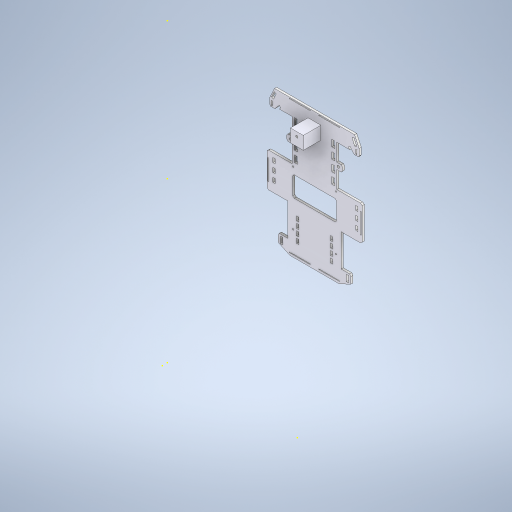
# Autodesk Inventor part: Robot_PMLD 1
Saved by Autodesk Inventor 2023 (Build 270158000, 158)
## iProperties
Created: 2025-05-12
Part Number: Robot_PMLD 1
Material: UHMW, White
Document SubType Name: Modeling
Designer: ASUS
Density: 0.94 g/cm^3
Appearance: Smooth - White
Author: ASUS
Autodesk Inventor part; units mm, degrees
ref_plane "YZ Plane" through (0, 0, 0) normal (1, 0, 0) x (0, 1, 0)
ref_plane "XZ Plane" through (0, 0, 0) normal (0, 1, 0) x (-1, 0, 0)
ref_plane "XY Plane" through (0, 0, 0) normal (0, 0, 1) x (1, 0, 0)
sketch "Sketch1" plane through (0, 0, 0) normal (0, 0, 1) x (1, 0, 0)
  line L0 (268.6934, 688.1739) -> (438.6934, 688.1739)
  line L1 (268.6934, 688.1739) -> (260.6934, 688.1739)
  line L2 (438.6934, 688.1739) -> (446.6934, 688.1739)
  line L3 (260.6934, 688.1739) -> (250.1279, 665.5162)
  line L4 (260.6934, 688.1739) -> (285.6934, 688.1739) construction
  line L5 (250.1279, 665.5162) -> (250.1279, 650.5162)
  line L6 (250.1279, 650.5162) -> (251.6279, 647.9181)
  line L7 (250.1279, 650.5162) -> (253.1279, 650.5162) construction
  line L8 (251.6279, 647.9181) -> (261.6279, 647.9181)
  line L9 (261.6279, 647.9181) -> (271.2697, 659.4088)
  line L10 (271.2697, 659.4088) -> (275.0999, 656.1948)
  line L11 (275.0999, 656.1948) -> (271.886, 652.3646)
  line L12 (271.886, 652.3646) -> (301.886, 652.3646)
  line L13 (446.6934, 688.1739) -> (457.2587, 665.5161)
  line L14 (457.2587, 665.5161) -> (457.2587, 650.5161)
  line L15 (457.2587, 650.5161) -> (455.7587, 647.9181)
  line L16 (455.7587, 647.9181) -> (445.7587, 647.9181)
  line L17 (445.7587, 647.9181) -> (436.117, 659.4088)
  line L18 (436.117, 659.4088) -> (432.2867, 656.1949)
  line L19 (432.2867, 656.1949) -> (435.5007, 652.3647)
  line L20 (435.5007, 652.3647) -> (405.5007, 652.3648)
  line L21 (301.886, 557.3687) -> (247.2816, 557.3687)
  line L22 (405.5007, 557.2878) -> (460.436, 557.2878)
  line L23 (460.436, 477.2878) -> (405.436, 477.2878)
  line L24 (405.436, 477.2878) -> (405.436, 402.2878)
  line L25 (301.6933, 402.3487) -> (271.6933, 402.3487)
  line L26 (405.436, 402.2878) -> (435.436, 402.2878)
  line L27 (435.436, 402.2878) -> (437.936, 397.9576)
  line L28 (437.936, 397.9576) -> (437.936, 382.9576)
  line L29 (271.6933, 402.3487) -> (276.6933, 402.3487) construction
  line L30 (269.3213, 397.9576) -> (269.3213, 382.9576)
  line L31 (269.3213, 382.9576) -> (296.5105, 370.2791)
  line L32 (437.936, 382.9576) -> (410.7467, 370.2791)
  line L33 (410.7467, 370.2791) -> (296.5105, 370.2791)
  line L34 (353.6934, 668.1738) -> (333.6934, 668.1738)
  line L35 (353.6934, 668.1738) -> (373.6934, 668.1738)
  line L36 (373.6934, 668.1738) -> (373.6934, 638.1738)
  line L37 (333.6934, 638.1738) -> (333.6934, 668.1738)
  line L38 (353.6934, 663.1738) -> (343.6934, 663.1738)
  line L39 (343.6934, 663.1738) -> (343.6934, 643.1738)
  line L40 (363.6934, 643.1738) -> (363.6934, 663.1738)
  line L41 (363.6934, 663.1738) -> (353.6934, 663.1738)
  line L42 (247.2816, 557.3687) -> (256.8212, 557.3687)
  line L43 (256.886, 547.3646) -> (261.886, 547.3646)
  line L44 (261.886, 547.3646) -> (261.886, 537.3646)
  line L45 (261.886, 537.3646) -> (256.886, 537.3646)
  line L46 (256.886, 537.3646) -> (256.886, 547.3646)
  line L47 (256.886, 527.3646) -> (261.886, 527.3646)
  line L48 (261.886, 527.3646) -> (261.886, 517.3646)
  line L49 (261.886, 517.3646) -> (256.886, 517.3646)
  line L50 (256.886, 517.3646) -> (256.886, 527.3646)
  line L51 (256.886, 507.3646) -> (261.886, 507.3646)
  line L52 (261.886, 507.3646) -> (261.886, 497.3646)
  line L53 (261.886, 497.3646) -> (256.886, 497.3646)
  line L54 (256.886, 497.3646) -> (256.886, 507.3646)
  line L55 (311.886, 457.3646) -> (316.886, 457.3646)
  line L56 (316.886, 457.3646) -> (316.886, 447.3646)
  line L57 (316.886, 447.3646) -> (311.886, 447.3646)
  line L58 (311.886, 447.3646) -> (311.886, 457.3646)
  line L59 (311.886, 442.3646) -> (316.886, 442.3646)
  line L60 (316.886, 442.3646) -> (316.886, 432.3646)
  line L61 (316.886, 432.3646) -> (311.886, 432.3646)
  line L62 (311.886, 432.3646) -> (311.886, 442.3646)
  line L63 (311.886, 427.3646) -> (316.886, 427.3646)
  line L64 (316.886, 427.3646) -> (316.886, 417.3646)
  line L65 (316.886, 417.3646) -> (311.886, 417.3646)
  line L66 (311.886, 417.3646) -> (311.886, 427.3646)
  line L67 (311.886, 412.3646) -> (316.886, 412.3646)
  line L68 (316.886, 412.3646) -> (316.886, 402.3646)
  line L69 (316.886, 402.3646) -> (311.886, 402.3646)
  line L70 (311.886, 402.3646) -> (311.886, 412.3646)
  line L71 (353.6286, 537.2874) -> (401.1286, 537.2874)
  line L72 (353.6286, 537.2874) -> (306.1286, 537.2874)
  line L73 (306.1286, 537.2874) -> (302.9146, 533.4572)
  line L74 (306.1286, 537.2874) -> (311.1286, 537.2874) construction
  line L75 (302.9146, 533.4572) -> (302.9146, 493.4572)
  line L76 (401.1286, 537.2874) -> (404.7816, 533.8734)
  line L77 (404.7816, 533.8734) -> (404.7816, 493.8734)
  line L78 (302.9146, 493.4572) -> (306.7497, 490.249)
  line L79 (306.7497, 490.249) -> (401.7497, 490.249)
  line L80 (401.7497, 490.249) -> (404.7816, 493.8734)
  line L81 (460.436, 557.2878) -> (450.436, 557.2878)
  line L82 (247.2816, 557.3687) -> (243.3598, 554.2673)
  line L83 (246.5737, 477.267) -> (243.3598, 481.0972)
  line L84 (246.5737, 477.267) -> (251.5737, 477.267) construction
  line L85 (243.3598, 481.0972) -> (243.3598, 554.2673)
  line L86 (460.436, 557.2878) -> (464.4205, 554.2673)
  line L87 (460.436, 477.2878) -> (464.2662, 480.5017)
  line L88 (460.436, 477.2878) -> (465.436, 477.2878) construction
  line L89 (464.2662, 480.5017) -> (464.4205, 554.2673)
  line L90 (454.4205, 547.2878) -> (449.4205, 547.2878)
  line L91 (449.4205, 547.2878) -> (449.4205, 537.2878)
  line L92 (449.4205, 537.2878) -> (454.4205, 537.2878)
  line L93 (454.4205, 537.2878) -> (454.4205, 547.2878)
  line L94 (454.4205, 527.2878) -> (449.4205, 527.2878)
  line L95 (449.4205, 527.2878) -> (449.4205, 517.2878)
  line L96 (449.4205, 517.2878) -> (454.4205, 517.2878)
  line L97 (454.4205, 517.2878) -> (454.4205, 527.2878)
  line L98 (454.4205, 507.2878) -> (449.4205, 507.2878)
  line L99 (449.4205, 507.2878) -> (449.4205, 497.2878)
  line L100 (449.4205, 497.2878) -> (454.4205, 497.2878)
  line L101 (454.4205, 497.2878) -> (454.4205, 507.2878)
  line L102 (306.886, 652.3646) -> (313.886, 652.3646)
  line L103 (313.886, 652.3646) -> (313.886, 637.3646)
  line L104 (313.886, 637.3646) -> (306.886, 637.3646)
  line L105 (306.886, 637.3646) -> (306.886, 652.3646)
  line L106 (306.886, 627.3646) -> (313.886, 627.3646)
  line L107 (313.886, 627.3646) -> (313.886, 612.3646)
  line L108 (313.886, 612.3646) -> (306.886, 612.3646)
  line L109 (306.886, 612.3646) -> (306.886, 627.3646)
  line L110 (306.886, 602.3646) -> (313.886, 602.3646)
  line L111 (313.886, 602.3646) -> (313.886, 587.3646)
  line L112 (313.886, 587.3646) -> (306.886, 587.3646)
  line L113 (306.886, 587.3646) -> (306.886, 602.3646)
  line L114 (306.886, 577.3646) -> (313.886, 577.3646)
  line L115 (313.886, 577.3646) -> (313.886, 562.3646)
  line L116 (313.886, 562.3646) -> (306.886, 562.3646)
  line L117 (306.886, 562.3646) -> (306.886, 577.3646)
  line L118 (400.5007, 652.3648) -> (393.5007, 652.3648)
  line L119 (393.5007, 652.3648) -> (393.5007, 637.3648)
  line L120 (393.5007, 637.3648) -> (400.5007, 637.3648)
  line L121 (400.5007, 637.3648) -> (400.5007, 652.3648)
  line L122 (400.5007, 627.3648) -> (393.5007, 627.3648)
  line L123 (393.5007, 627.3648) -> (393.5007, 612.3648)
  line L124 (393.5007, 612.3648) -> (400.5007, 612.3648)
  line L125 (400.5007, 612.3648) -> (400.5007, 627.3648)
  line L126 (400.5007, 602.3648) -> (393.5007, 602.3648)
  line L127 (393.5007, 602.3648) -> (393.5007, 587.3648)
  line L128 (393.5007, 587.3648) -> (400.5007, 587.3648)
  line L129 (400.5007, 587.3648) -> (400.5007, 602.3648)
  line L130 (400.5007, 577.3648) -> (393.5007, 577.3648)
  line L131 (393.5007, 577.3648) -> (393.5007, 562.3648)
  line L132 (393.5007, 562.3648) -> (400.5007, 562.3648)
  line L133 (400.5007, 562.3648) -> (400.5007, 577.3648)
  line L134 (250.1279, 665.5162) -> (255.1279, 665.5162) construction
  line L135 (253.1279, 650.5162) -> (256.1279, 650.5162)
  line L136 (256.1279, 650.5162) -> (256.1279, 660.5162)
  line L137 (256.1279, 660.5162) -> (253.1279, 660.5162)
  line L138 (253.1279, 660.5162) -> (253.1279, 650.5162)
  line L139 (452.2587, 650.5161) -> (449.2587, 650.5161)
  line L140 (449.2587, 650.5161) -> (449.2587, 660.5161)
  line L141 (449.2587, 660.5161) -> (452.2587, 660.5161)
  line L142 (452.2587, 660.5161) -> (452.2587, 650.5161)
  line L143 (258.3995, 665.5162) -> (263.3995, 665.5162) construction
  line L144 (446.991, 665.5162) -> (451.5445, 667.5814)
  line L145 (446.991, 665.5162) -> (451.5445, 667.5814)
  line L146 (451.5445, 667.5814) -> (445.3487, 681.242)
  line L147 (445.3487, 681.242) -> (440.7952, 679.1768)
  line L148 (440.7952, 679.1768) -> (446.991, 665.5162)
  line L149 (258.3995, 665.5162) -> (253.868, 667.6293)
  line L150 (258.3995, 665.5162) -> (263.3995, 665.5162) construction
  line L151 (258.3995, 665.5162) -> (253.868, 667.6293)
  line L152 (253.868, 667.6293) -> (260.2072, 681.2239)
  line L153 (260.2072, 681.2239) -> (264.7388, 679.1108)
  line L154 (264.7388, 679.1108) -> (258.3995, 665.5162)
  line L155 (269.3213, 397.9576) -> (271.6933, 402.3487)
  line L156 (274.3213, 382.9576) -> (274.3213, 397.9576)
  line L157 (274.3213, 397.9576) -> (279.3213, 397.9576)
  line L158 (279.3213, 397.9576) -> (279.3213, 382.9576)
  line L159 (279.3213, 382.9576) -> (274.3213, 382.9576)
  line L160 (432.936, 382.9576) -> (432.936, 397.9576)
  line L161 (432.936, 397.9576) -> (427.936, 397.9576)
  line L162 (427.936, 397.9576) -> (427.936, 382.9576)
  line L163 (427.936, 382.9576) -> (432.936, 382.9576)
  line L164 (343.6286, 375.2791) -> (313.6286, 375.2791)
  line L165 (313.6286, 375.2791) -> (313.6286, 380.2791)
  line L166 (313.6286, 380.2791) -> (343.6286, 380.2791)
  line L167 (343.6286, 380.2791) -> (343.6286, 375.2791)
  line L168 (363.6286, 375.2791) -> (393.6286, 375.2791)
  line L169 (393.6286, 375.2791) -> (393.6286, 380.2791)
  line L170 (393.6286, 380.2791) -> (363.6286, 380.2791)
  line L171 (363.6286, 380.2791) -> (363.6286, 375.2791)
  line L172 (301.886, 652.3646) -> (301.886, 612.3646)
  line L173 (301.886, 557.3687) -> (301.886, 597.3687)
  line L174 (301.886, 612.3646) -> (291.886, 612.3646)
  line L175 (301.886, 597.3687) -> (291.886, 597.3687)
  arc A0 (291.886, 612.3646) -> (291.886, 597.3687) centre (298.5027, 604.8667) ccw
  circle A1 centre (298.5027, 604.8667) radius 3
  line L176 (405.5007, 652.3648) -> (405.5007, 612.3648)
  line L177 (405.5007, 557.2878) -> (405.5007, 597.2878)
  line L178 (405.5007, 612.3648) -> (415.5007, 612.3648)
  line L179 (405.5007, 597.2878) -> (415.5007, 597.2878)
  arc A2 (415.5007, 597.2878) -> (415.5007, 612.3648) centre (408.9302, 604.8263) ccw
  circle A3 centre (408.9302, 604.8263) radius 3
  line L180 (301.6933, 402.3487) -> (301.6933, 477.3487)
  line L181 (301.6933, 477.3487) -> (246.5737, 477.267)
  line L182 (395.436, 457.2878) -> (390.436, 457.2878)
  line L183 (390.436, 457.2878) -> (390.436, 447.2878)
  line L184 (390.436, 447.2878) -> (395.436, 447.2878)
  line L185 (395.436, 447.2878) -> (395.436, 457.2878)
  line L186 (395.436, 442.2878) -> (390.436, 442.2878)
  line L187 (390.436, 442.2878) -> (390.436, 432.2878)
  line L188 (390.436, 432.2878) -> (395.436, 432.2878)
  line L189 (395.436, 432.2878) -> (395.436, 442.2878)
  line L190 (395.436, 427.2878) -> (390.436, 427.2878)
  line L191 (390.436, 427.2878) -> (390.436, 417.2878)
  line L192 (390.436, 417.2878) -> (395.436, 417.2878)
  line L193 (395.436, 417.2878) -> (395.436, 427.2878)
  line L194 (395.436, 412.2878) -> (390.436, 412.2878)
  line L195 (390.436, 412.2878) -> (390.436, 402.2878)
  line L196 (390.436, 402.2878) -> (395.436, 402.2878)
  line L197 (395.436, 402.2878) -> (395.436, 412.2878)
  line L198 (343.6934, 643.1738) -> (343.6934, 638.1738)
  line L199 (363.6934, 643.1738) -> (363.6934, 638.1738)
  line L200 (333.6934, 638.1738) -> (343.6934, 638.1738)
  line L201 (363.6934, 638.1738) -> (373.6934, 638.1738)
  line L202 (401.7497, 490.249) -> (398.7497, 490.249)
  line L203 (306.7497, 490.249) -> (309.7497, 490.249)
  circle A4 centre (403.2657, 467.0612) radius 1.6
  circle A5 centre (303.4357, 467.0612) radius 1.6
  circle A6 centre (303.4357, 593.0112) radius 1.6
  circle A7 centre (403.2657, 593.0112) radius 1.6
  point P0 (0, 0)
  dimension "d0" = 170
  dimension "d1" = 8
  dimension "d2" = 8
  dimension "d3" = 25
  dimension "d4" = 115
  dimension "d5" = 15
  dimension "d11" = 3
  dimension "d12" = 60
  dimension "d13" = 10
  dimension "d14" = 15
  dimension "d15" = 130
  dimension "d16" = 5
  dimension "d17" = 5
  dimension "d19" = 30
  dimension "d22" = 25
  dimension "d23" = 15
  dimension "d27" = 3
  dimension "d28" = 10
  dimension "d29" = 15
  dimension "d30" = 130
  dimension "d31" = 5
  dimension "d32" = 5
  dimension "d33" = 30
  dimension "d47" = 55
  dimension "d51" = 75
  dimension "d52" = 30
  dimension "d53" = 30
  dimension "d54" = 5
  dimension "d55" = 120
  dimension "d56" = 15
  dimension "d59" = 15
  dimension "d60" = 30
  dimension "d61" = 115
  dimension "d62" = 30
  dimension "d75" = 30
  dimension "d76" = 40
  dimension "d77" = 5
  dimension "d78" = 10
  dimension "d79" = 20
  dimension "d81" = 20
  dimension "d82" = 10
  dimension "d100" = 5
  dimension "d101" = 10
  dimension "d103" = 5
  dimension "d104" = 10
  dimension "d106" = 5
  dimension "d107" = 10
  dimension "d113" = 5
  dimension "d114" = 10
  dimension "d116" = 5
  dimension "d117" = 10
  dimension "d119" = 5
  dimension "d120" = 10
  dimension "d122" = 5
  dimension "d123" = 10
  dimension "d139" = 5
  dimension "d140" = 130
  dimension "d141" = 40
  dimension "d142" = 5
  dimension "d143" = 40
  dimension "d144" = 5
  dimension "d145" = 95
  dimension "d147" = 5
  dimension "d148" = 5
  constraints: 408 end point, 61 parallel, 54 horizontal, 38 perpendicular, 8 centre point, 8 vertical, 7 point on line, 6 equal length, 4 point on circle, 3 collinear, 2 coincident
  measures "d0" distance of L0.start L0.end
  measures "d1" distance of L0.start L1.end
  measures "d2" distance of L0.end L2.end
  measures "d3" distance of L1.end L3.end
  measures "d4" angle of L3 L4
  measures "d5" distance of L3.end L5.end
  measures "d11" distance of L5.end L6.end
  measures "d12" angle of L6 L7
  measures "d13" distance of L6.end L8.end
  measures "d14" distance of L8.end L9.end
  measures "d15" angle of L9 L8
  measures "d16" distance of L9.end L10.end
  measures "d17" distance of L10.end L11.end
  measures "d19" distance of L11.end L12.end
  measures "d22" distance of L2.end L13.end
  measures "d23" distance of L13.end L14.end
  measures "d27" distance of L14.end L15.end
  measures "d28" distance of L15.end L16.end
  measures "d29" distance of L16.end L17.end
  measures "d30" angle of L16 L17
  measures "d31" distance of L17.end L18.end
  measures "d32" distance of L18.end L19.end
  measures "d33" distance of L19.end L20.end
  measures "d47" distance of L23.start L23.end
  measures "d51" distance of L23.end L24.end
  measures "d52" distance of L25.start L25.end
  measures "d53" distance of L24.end L26.end
  measures "d54" distance of L26.end L27.end
  measures "d55" angle of L26 L27
  measures "d56" distance of L27.end L28.end
  measures "d59" distance of L30.start L30.end
  measures "d60" distance of L30.end L31.end
  measures "d61" angle of L31 L30
  measures "d62" distance of L28.end L32.end
  measures "d75" distance of L35.end L36.end
  measures "d76" distance of L36.end L37.start
  measures "d77" distance of L34.start L38.start
  measures "d78" distance of L38.start L38.end
  measures "d79" distance of L38.end L39.end
  measures "d81" distance of L40.start L40.end
  measures "d82" distance of L40.end L38.start
  measures "d100" distance of L44.end L45.end
  measures "d101" distance of L43.end L44.end
  measures "d103" distance of L48.end L49.end
  measures "d104" distance of L47.end L48.end
  measures "d106" distance of L52.end L53.end
  measures "d107" distance of L51.end L52.end
  measures "d113" distance of L56.end L57.end
  measures "d114" distance of L55.end L56.end
  measures "d116" distance of L60.end L61.end
  measures "d117" distance of L59.end L60.end
  measures "d119" distance of L64.end L65.end
  measures "d120" distance of L63.end L64.end
  measures "d122" distance of L68.end L69.end
  measures "d123" distance of L67.end L68.end
  measures "d139" distance of L72.end L73.end
  measures "d140" angle of L73 L74
  measures "d141" distance of L73.end L75.end
  measures "d142" distance of L71.end L76.end
  measures "d143" distance of L76.end L77.end
  measures "d144" distance of L75.end L78.end
  measures "d145" distance of L78.end L79.end
  measures "d147" distance of L21.end L82.end
  measures "d148" distance of L83.start L83.end
sketch "Sketch2" plane through (0, 0, 0) normal (0, 0, 1) x (1, 0, 0)
  point P0 (0, 0)
sketch "Sketch5" plane through (0, 0, 0) normal (0, 0, 1) x (1, 0, 0)
  point P0 (0, 0)
extrude "Extrusion5" add sketch "Sketch1" along normal blind 50 contours L35 L36 L201 L199 L40 L41 L38 L39 L198 L200 L37 L34
extrude "Extrusion6" add sketch "Sketch1" along normal blind 12 contours L0 L2 L13 L14 L15 L16 L17 L18 L19 L20 L176 L178 A2 L179 L177 L22 L86 L89 L87 L23 L24 L26 L27 L28 L32 L33 L31 L30 L155 L25 L180 L181 L83 L85 L82 L21 L173 A6 L175 A0 L174 L172 L12 L11 L10 L9 L8 L6 L5 L3 L1 | A6 L173 | A4 | A5 | A7 picked at (302.9218, 592.6447)
sketch "Sketch13" plane through (0, 0, 12) normal (0, 0, 1) x (1, 0, 0)
  point P0 (0, 0)
sketch "Sketch14" plane through (0, 0, 12) normal (0, 0, 1) x (1, 0, 0)
  point P0 (0, 0)
sketch "Sketch15" plane through (0, 0, 12) normal (0, 0, 1) x (1, 0, 0)
  point P0 (0, 0)
sketch "Sketch16" plane through (301.886, 557.3687, 0) normal (-1, 0, 0) x (0, 0, 1)
  point P0 (0, -557.3687)
sketch "Sketch17" plane through (0, 0, 12) normal (0, 0, 1) x (1, 0, 0)
  point P0 (0, 0)
thread "Thread1" size "M6x1" class "6H" standard "ANSI Metric M Profile" length 43.6
thread "Thread2" size "M6x1" class "6H" standard "ANSI Metric M Profile" length 43.6
sketch "Sketch18" plane through (0, 0, 12) normal (0, 0, 1) x (1, 0, 0)
  point P0 (0, 0)
sketch "Sketch19" plane through (0, 0, 12) normal (0, 0, 1) x (1, 0, 0)
  point P0 (0, 0)
sketch "Sketch24" plane through (301.6933, 402.3487, 0) normal (-1, 0, 0) x (0, 0, 1)
  point P0 (0, -402.3487)
sketch "Sketch26" plane through (301.6933, 402.3487, 0) normal (-1, 0, 0) x (0, 0, 1)
  point P0 (0, -402.3487)
sketch "Sketch27" plane through (301.6933, 477.3487, 0) normal (0.0014818, -0.9999989, 0) x (0.9999989, 0.0014818, 0)
  line L0 (0, 0) -> (-0.1111, 0) projected
  line L1 (0, 0) -> (-10, 0)
  line L2 (-55.1196, 0) -> (0, 0) projected
  line L3 (-10, 0) -> (-10, 12)
  line L4 (100.0754, 0) -> (5.0755, 0) projected
  line L5 (-10, 0) -> (2, 0) construction
  line L6 (-55.1196, 12) -> (0, 12) projected
  line L7 (-10, 12) -> (0, 12)
  line L8 (0, 12) -> (0, 0)
  point P0 (-302.4003, 0)
  dimension "d332" = 10
  dimension "d333" = 12
  dimension "d334" = 90
  dimension "d335" = 10
  dimension "d336" = 12
  constraints: 10 end point, 2 perpendicular, 1 horizontal, 1 point on line
  measures "d332" distance of L0.start L1.end
  measures "d333" distance of L1.end L3.end
  measures "d334" angle of L5 L3
  measures "d335" distance of L3.end L6.end
  measures "d336" distance of L6.end L0.start
extrude "Extrusion16" add sketch "Sketch27" along normal blind 75
sketch "Sketch28" plane through (405.436, 477.2878, 0) normal (0, -1, 0) x (1, 0, 0)
  line L0 (0, 0) -> (0, 12) projected
  line L1 (0, 0) -> (10, 0)
  line L2 (0, 0) -> (55, 0) projected
  line L3 (10, 0) -> (10, 12)
  line L4 (0, 12) -> (55, 12) projected
  line L5 (10, 12) -> (0, 12)
  line L6 (0, 12) -> (0, 0)
  point P0 (-405.436, 0)
  dimension "d339" = 10
  dimension "d340" = 12
  dimension "d341" = 90
  dimension "d342" = 10
  dimension "d343" = 12
  constraints: 8 end point, 2 perpendicular, 1 point on line
  measures "d339" distance of L0.start L1.end
  measures "d340" distance of L1.end L3.end
  measures "d341" angle of L3 L1
  measures "d342" distance of L3.end L5.end
  measures "d343" distance of L5.end L0.start
extrude "Extrusion17" add sketch "Sketch28" along normal blind 75
sketch "Sketch29" plane through (0, 0, 12) normal (0, 0, 1) x (1, 0, 0)
  point P0 (0, 0)
sketch "Sketch30" plane through (0, 0, 12) normal (0, 0, 1) x (1, 0, 0)
  line L0 (302.9146, 533.4572) -> (306.1286, 537.2874) projected
  line L1 (306.1286, 537.2874) -> (401.1286, 537.2874) projected
  circle A0 centre (303.7136, 552.2874) radius 1.6
  circle A1 centre (403.5436, 552.2874) radius 1.6
  line L2 (405.5007, 557.2878) -> (405.5007, 597.2878) projected
  circle A2 centre (403.5436, 426.3374) radius 1.6
  circle A3 centre (303.7136, 426.3374) radius 1.6
  point P0 (0, 0)
  dimension "d351" = 3.2
  dimension "d352" = 3.2
  dimension "d355" = 3.2
  dimension "d357" = 3.2
  constraints: 4 centre point
  measures "d351" diameter of A0
  measures "d352" diameter of A1
  measures "d355" diameter of A2
  measures "d357" diameter of A3
extrude "Extrusion18" cut sketch "Sketch30" against normal blind 20 contours A3
extrude "Extrusion19" cut sketch "Sketch30" against normal blind 20 contours A2
extrude "Extrusion20" cut sketch "Sketch30" against normal blind 20 contours A1
extrude "Extrusion21" cut sketch "Sketch30" against normal blind 20 contours A0
thread "Thread7" size "M3.5x0.6" class "6H" standard "ANSI Metric M Profile" length 43.6
thread "Thread8" size "M3.5x0.6" class "6H" standard "ANSI Metric M Profile" length 43.6
thread "Thread9" size "M3.5x0.6" class "6H" standard "ANSI Metric M Profile" length 43.6
thread "Thread10" size "M3.5x0.6" class "6H" standard "ANSI Metric M Profile" length 43.6
sketch "Sketch31" plane through (0, 0, 50) normal (0, 0, 1) x (1, 0, 0)
  line L0 (333.6934, 638.1738) -> (343.6934, 638.1738) projected
  line L1 (333.6934, 668.1738) -> (333.6934, 638.1738) projected
  line L2 (333.6934, 638.1738) -> (333.6934, 668.1738)
  line L3 (373.6934, 668.1738) -> (333.6934, 668.1738) projected
  line L4 (333.6934, 668.1738) -> (373.6934, 668.1738)
  line L5 (373.6934, 638.1738) -> (373.6934, 668.1738) projected
  line L6 (373.6934, 668.1738) -> (373.6934, 638.1738)
  line L7 (373.6934, 638.1738) -> (333.6934, 638.1738)
  point P0 (0, 0)
  dimension "d374" = 30
  dimension "d375" = 40
  dimension "d376" = 30
  dimension "d377" = 40
  constraints: 8 end point, 2 collinear, 2 perpendicular
  measures "d374" distance of L0.start L1.start
  measures "d375" distance of L1.start L3.start
  measures "d376" distance of L3.start L5.start
  measures "d377" distance of L5.start L0.start
extrude "Extrusion22" add sketch "Sketch31" along normal blind 3
sketch "Sketch32" plane through (0, 0, 53) normal (0, 0, 1) x (1, 0, 0)
  line L0 (373.6934, 668.1738) -> (333.6934, 668.1738) projected
  circle A0 centre (353.6934, 658.1738) radius 2.5
  point P0 (0, 0)
  dimension "d381" = 5
  constraints: 1 centre point
  measures "d381" diameter of A0
extrude "Extrusion23" cut sketch "Sketch32" against normal blind 2
thread "Thread11" size "M5x0.8" class "6H" standard "ANSI Metric M Profile" length 43.6
sketch "Sketch33" plane through (0, 0, 12) normal (0, 0, 1) x (1, 0, 0)
  line L0 (296.5105, 370.2791) -> (410.7467, 370.2791) projected
  line L1 (313.6286, 375.2791) -> (313.6286, 380.2791) projected
  line L2 (313.6286, 375.2791) -> (295.6286, 375.2791)
  line L3 (295.6286, 375.2791) -> (295.6286, 380.2791)
  line L4 (295.6286, 380.2791) -> (313.6286, 380.2791)
  line L5 (393.6286, 380.2791) -> (393.6286, 375.2791) projected
  line L6 (393.6286, 380.2791) -> (411.6286, 380.2791)
  line L7 (411.6286, 380.2791) -> (411.6286, 375.2791)
  line L8 (411.6286, 375.2791) -> (393.6286, 375.2791)
  point P0 (0, 0)
  dimension "d388" = 18
  dimension "d389" = 5
  dimension "d390" = 18
  dimension "d391" = 5
  dimension "d392" = 18
  constraints: 12 end point, 2 horizontal, 1 perpendicular, 1 vertical
  measures "d388" distance of L1.start L2.end
  measures "d389" distance of L2.end L3.end
  measures "d390" distance of L5.start L6.end
  measures "d391" distance of L6.end L7.end
  measures "d392" distance of L7.end L5.end
extrude "Extrusion24" cut sketch "Sketch33" against normal blind 20 contours L2 L3 L4 L1
extrude "Extrusion25" cut sketch "Sketch33" against normal blind 20 contours L6 L7 L8 L5
sketch "Sketch34" plane through (0, 0, 12) normal (0, 0, 1) x (1, 0, 0)
  point P0 (0, 0)
sketch "Sketch35" plane through (0, 0, 12) normal (0, 0, 1) x (1, 0, 0)
  line L0 (343.6286, 380.2791) -> (343.6286, 375.2791) projected
  line L1 (343.6286, 375.2791) -> (343.6286, 376.7791)
  line L2 (343.6286, 376.7791) -> (295.6286, 376.7791)
  line L3 (295.6286, 380.2791) -> (295.6286, 375.2791) projected
  line L4 (295.6286, 376.7791) -> (295.6286, 380.2791)
  line L5 (295.6286, 380.2791) -> (343.6286, 380.2791) projected
  line L6 (295.6286, 380.2791) -> (343.6286, 380.2791)
  line L7 (343.6286, 380.2791) -> (343.6286, 376.7791)
  line L8 (411.6286, 375.2791) -> (363.6286, 375.2791) projected
  line L9 (411.6286, 375.2791) -> (411.6286, 376.7791)
  line L10 (411.6286, 380.2791) -> (411.6286, 375.2791) projected
  line L11 (411.6286, 376.7791) -> (363.6286, 376.7791)
  line L12 (363.6286, 380.2791) -> (411.6286, 380.2791) projected
  line L13 (363.6286, 376.7791) -> (363.6286, 380.2791)
  line L14 (363.6286, 380.2791) -> (411.6286, 380.2791)
  line L15 (411.6286, 380.2791) -> (411.6286, 376.7791)
  point P0 (0, 0)
  dimension "d397" = 1.5
  dimension "d398" = 48
  dimension "d399" = 3.5
  dimension "d400" = 48
  dimension "d401" = 3.5
  dimension "d402" = 1.5
  dimension "d403" = 48
  dimension "d404" = 3.5
  dimension "d405" = 48
  dimension "d406" = 3.5
  constraints: 20 end point, 4 perpendicular, 2 collinear, 2 point on line
  measures "d397" distance of L0.end L1.end
  measures "d398" distance of L1.end L2.end
  measures "d399" distance of L2.end L3.start
  measures "d400" distance of L3.start L0.start
  measures "d401" distance of L0.start L1.end
  measures "d402" distance of L8.start L9.end
  measures "d403" distance of L9.end L11.end
  measures "d404" distance of L11.end L12.start
  measures "d405" distance of L12.start L10.start
  measures "d406" distance of L10.start L9.end
sketch "Sketch36" plane through (296.5105, 370.2791, 0) normal (0, -1, 0) x (1, 0, 0)
  point P0 (-296.5105, 0)
extrude "Extrusion26" add sketch "Sketch35" against normal blind 12 contours L0 L2 L3 L5
extrude "Extrusion27" add sketch "Sketch35" against normal blind 12 contours L10 L11 L13 L12
sketch "Sketch37" plane through (0, 0, 12) normal (0, 0, 1) x (1, 0, 0)
  line L0 (446.6934, 688.1739) -> (260.6934, 688.1739) projected
  line L1 (343.6934, 686.1739) -> (295.6934, 686.1739)
  line L2 (295.6934, 686.1739) -> (295.6934, 684.6739)
  line L3 (295.6934, 684.6739) -> (343.6934, 684.6739)
  line L4 (343.6934, 684.6739) -> (343.6934, 686.1739)
  line L5 (363.6934, 686.1739) -> (411.6934, 686.1739)
  line L6 (411.6934, 686.1739) -> (411.6934, 684.6739)
  line L7 (411.6934, 684.6739) -> (363.6934, 684.6739)
  line L8 (363.6934, 684.6739) -> (363.6934, 686.1739)
  point P0 (0, 0)
  dimension "d415" = 48
  dimension "d416" = 1.5
  dimension "d417" = 48
  dimension "d418" = 1.5
  dimension "d420" = 48
  dimension "d421" = 1.5
  dimension "d422" = 48
  dimension "d423" = 1.5
  constraints: 16 end point, 2 horizontal, 2 parallel, 1 perpendicular, 1 vertical
  measures "d415" distance of L1.start L1.end
  measures "d416" distance of L1.end L2.end
  measures "d417" distance of L2.end L3.end
  measures "d418" distance of L3.end L1.start
  measures "d420" distance of L5.start L5.end
  measures "d421" distance of L5.end L6.end
  measures "d422" distance of L6.end L7.end
  measures "d423" distance of L7.end L5.start
extrude "Extrusion28" cut sketch "Sketch37" against normal blind 12 contours L4 L3 L2 L1
extrude "Extrusion29" cut sketch "Sketch37" against normal blind 12 contours L5 L6 L7 L8
sketch "Sketch38" plane through (0, 0, 12) normal (0, 0, 1) x (1, 0, 0)
  line L0 (243.3598, 554.2673) -> (243.3598, 481.0972) projected
  line L1 (245.3598, 517.6823) -> (245.3598, 541.6823)
  line L2 (245.3598, 541.6823) -> (246.8598, 541.6823)
  line L3 (246.8598, 541.6823) -> (246.8598, 493.6823)
  line L4 (246.8598, 493.6823) -> (245.3598, 493.6823)
  line L5 (245.3598, 493.6823) -> (245.3598, 517.6823)
  point P0 (0, 0)
  dimension "d429" = 24
  dimension "d430" = 1.5
  dimension "d431" = 48
  dimension "d432" = 1.5
  dimension "d433" = 24
  constraints: 10 end point, 2 perpendicular, 1 collinear, 1 point on line
  measures "d429" distance of L1.start L1.end
  measures "d430" distance of L1.end L2.end
  measures "d431" distance of L2.end L3.end
  measures "d432" distance of L3.end L4.end
  measures "d433" distance of L4.end L1.start
extrude "Extrusion30" cut sketch "Sketch38" against normal blind 12
sketch "Sketch39" plane through (0, 0, 12) normal (0, 0, 1) x (1, 0, 0)
  line L0 (464.2662, 480.5017) -> (464.4205, 554.2673) projected
  line L1 (462.3434, 517.3845) -> (462.3434, 541.3845)
  line L2 (462.3434, 541.3845) -> (460.8434, 541.3845)
  line L3 (460.8434, 541.3845) -> (460.8434, 493.3845)
  line L4 (460.8434, 493.3845) -> (462.3434, 493.3845)
  line L5 (462.3434, 493.3845) -> (462.3434, 517.3845)
  point P0 (0, 0)
  dimension "d437" = 24
  dimension "d438" = 1.5
  dimension "d439" = 48
  dimension "d440" = 1.5
  dimension "d441" = 24
  constraints: 10 end point, 2 perpendicular, 1 point on line
  measures "d437" distance of L1.start L1.end
  measures "d438" distance of L1.end L2.end
  measures "d439" distance of L2.end L3.end
  measures "d440" distance of L3.end L4.end
  measures "d441" distance of L4.end L1.start
extrude "Extrusion31" cut sketch "Sketch39" against normal blind 12
sketch "Sketch40" plane through (333.6934, 668.1738, 12) normal (0, 1, 0) x (1, 0, 0)
  line L0 (40, 0) -> (40, -41) projected
  line L1 (78, 0) -> (30, 0) projected
  line L2 (40, -41) -> (38, -41)
  line L3 (38, -41) -> (38, 0)
  line L4 (38, 0) -> (40, 0)
  line L5 (40, 0) -> (40, -41)
  line L6 (0, 0) -> (0, -41) projected
  line L7 (10, 0) -> (-38, 0) projected
  line L8 (0, -41) -> (2, -41)
  line L9 (2, -41) -> (2, 0)
  line L10 (2, 0) -> (0, 0)
  line L11 (0, 0) -> (0, -41)
  point P0 (-333.6934, 12)
  dimension "d444" = 2
  dimension "d445" = 2
  constraints: 16 end point, 4 parallel, 2 horizontal, 2 perpendicular, 2 point on line
  measures "d444" distance of L3.end L4.end
  measures "d445" distance of L10.end L9.end
extrude "Extrusion32" cut sketch "Sketch40" against normal blind 100
sketch "Sketch41" plane through (335.6934, 668.1738, 53) normal (0, 1, 0) x (1, 0, 0)
  line L0 (36, 0) -> (36, 41) projected
  line L1 (111, 41) -> (-75, 41) projected
  line L2 (36, 0) -> (33, 0)
  line L3 (33, 0) -> (33, 41)
  line L4 (33, 41) -> (36, 41)
  line L5 (36, 41) -> (36, 0)
  line L6 (0, 41) -> (0, 0) projected
  line L7 (0, 0) -> (3, 0)
  line L8 (3, 0) -> (3, 41)
  line L9 (3, 41) -> (0, 41)
  line L10 (0, 41) -> (0, 0)
  point P0 (-335.6934, 53)
  point P1 (3, 41)
  dimension "d448" = 3
  dimension "d449" = 3
  constraints: 16 end point, 4 parallel, 2 horizontal, 2 perpendicular, 2 point on line
  measures "d448" distance of L3.end L4.end
  measures "d449" distance of L9.end L8.end
extrude "Extrusion33" cut sketch "Sketch41" against normal blind 100
sketch "Sketch42" plane through (0, 0, 12) normal (0, 0, 1) x (1, 0, 0)
  point P0 (0, 0)
sketch "Sketch43" plane through (260.6934, 688.1739, 0) normal (0, 1, 0) x (1, 0, 0)
  point P0 (-260.6934, 0)
sketch "Sketch44" plane through (0, 0, 0) normal (0, 0, -1) x (-1, 0, 0)
  line L0 (-446.6934, 688.1739) -> (-260.6934, 688.1739) projected
  line L1 (-446.6934, 688.1739) -> (-260.6934, 688.1739)
  line L2 (-250.1279, 665.5162) -> (-250.1279, 650.5162) projected
  line L3 (-260.6934, 688.1739) -> (-250.1279, 665.5162)
  line L4 (-250.1279, 665.5162) -> (-250.1279, 650.5162)
  line L5 (-250.1279, 650.5162) -> (-251.6279, 647.9181) projected
  line L6 (-250.1279, 650.5162) -> (-251.6279, 647.9181)
  line L7 (-261.6279, 647.9181) -> (-271.2697, 659.4088) projected
  line L8 (-251.6279, 647.9181) -> (-261.6279, 647.9181)
  line L9 (-261.6279, 647.9181) -> (-271.2697, 659.4088)
  line L10 (-275.0999, 656.1948) -> (-271.886, 652.3646) projected
  line L11 (-271.2697, 659.4088) -> (-275.0999, 656.1948)
  line L12 (-275.0999, 656.1948) -> (-271.886, 652.3646)
  line L13 (-271.886, 652.3646) -> (-301.886, 652.3646) projected
  line L14 (-271.886, 652.3646) -> (-301.886, 652.3646)
  line L15 (-301.886, 652.3646) -> (-301.886, 612.3646) projected
  line L16 (-301.886, 652.3646) -> (-301.886, 612.3646)
  line L17 (-301.886, 612.3646) -> (-291.886, 612.3646) projected
  line L18 (-301.886, 612.3646) -> (-291.886, 612.3646)
  line L19 (-291.886, 597.3687) -> (-301.886, 597.3687) projected
  arc A0 (-291.886, 597.3687) -> (-291.886, 612.3646) centre (-298.5027, 604.8667) ccw
  line L20 (-291.886, 597.3687) -> (-301.886, 597.3687)
  line L21 (-301.886, 557.3687) -> (-247.2816, 557.3687) projected
  line L22 (-301.886, 597.3687) -> (-301.886, 557.3687)
  line L23 (-457.2587, 665.5161) -> (-446.6934, 688.1739) projected
  line L24 (-446.6934, 688.1739) -> (-457.2587, 665.5161)
  line L25 (-457.2587, 650.5161) -> (-457.2587, 665.5161) projected
  line L26 (-457.2587, 665.5161) -> (-457.2587, 650.5161)
  line L27 (-445.7587, 647.9181) -> (-455.7587, 647.9181) projected
  line L28 (-457.2587, 650.5161) -> (-455.7587, 647.9181)
  line L29 (-455.7587, 647.9181) -> (-445.7587, 647.9181)
  line L30 (-432.2867, 656.1949) -> (-436.117, 659.4088) projected
  line L31 (-445.7587, 647.9181) -> (-436.117, 659.4088)
  line L32 (-436.117, 659.4088) -> (-432.2867, 656.1949)
  line L33 (-405.5007, 652.3648) -> (-435.5007, 652.3647) projected
  line L34 (-432.2867, 656.1949) -> (-435.5007, 652.3647)
  line L35 (-435.5007, 652.3647) -> (-405.5007, 652.3647)
  line L36 (-405.5007, 612.3648) -> (-405.5007, 652.3648) projected
  line L37 (-405.5007, 652.3647) -> (-405.5007, 612.3647)
  line L38 (-405.5007, 612.3647) -> (-415.5007, 612.3648)
  line L39 (-415.5007, 612.3648) -> (-405.5007, 612.3648) projected
  line L40 (-405.5007, 597.2878) -> (-415.5007, 597.2878) projected
  arc A1 (-415.5007, 612.3648) -> (-415.5007, 597.2878) centre (-408.9302, 604.8263) ccw
  line L41 (-415.5007, 597.2878) -> (-405.5007, 597.2878)
  line L42 (-405.5007, 557.2878) -> (-405.5007, 597.2878) projected
  line L43 (-405.5007, 597.2878) -> (-405.5007, 557.2878)
  line L44 (-464.4205, 554.2673) -> (-460.436, 557.2878) projected
  line L45 (-405.5007, 557.2878) -> (-460.436, 557.2878)
  line L46 (-460.436, 557.2878) -> (-464.4205, 554.2673)
  line L47 (-460.436, 477.2878) -> (-464.2662, 480.5017) projected
  line L48 (-464.4205, 554.2673) -> (-464.2662, 480.5017)
  line L49 (-464.2662, 480.5017) -> (-460.436, 477.2878)
  line L50 (-415.436, 477.2878) -> (-415.436, 402.2878) projected
  line L51 (-460.436, 477.2878) -> (-415.436, 477.2878)
  line L52 (-415.436, 477.2878) -> (-415.436, 402.2878)
  line L53 (-435.436, 402.2878) -> (-415.436, 402.2878) projected
  line L54 (-415.436, 402.2878) -> (-435.436, 402.2878)
  line L55 (-437.936, 397.9576) -> (-435.436, 402.2878) projected
  line L56 (-435.436, 402.2878) -> (-437.936, 397.9576)
  line L57 (-437.936, 382.9576) -> (-437.936, 397.9576) projected
  line L58 (-437.936, 397.9576) -> (-437.936, 382.9576)
  line L59 (-296.5105, 370.2791) -> (-410.7467, 370.2791) projected
  line L60 (-437.936, 382.9576) -> (-410.7467, 370.2791)
  line L61 (-269.3213, 382.9576) -> (-296.5105, 370.2791) projected
  line L62 (-410.7467, 370.2791) -> (-296.5105, 370.2791)
  line L63 (-269.3213, 397.9576) -> (-269.3213, 382.9576) projected
  line L64 (-296.5105, 370.2791) -> (-269.3213, 382.9576)
  line L65 (-269.3213, 382.9576) -> (-269.3213, 397.9576)
  line L66 (-271.6933, 402.3487) -> (-269.3213, 397.9576) projected
  line L67 (-269.3213, 397.9576) -> (-271.6933, 402.3487)
  line L68 (-291.8044, 402.3487) -> (-271.6933, 402.3487) projected
  line L69 (-271.6933, 402.3487) -> (-291.8044, 402.3487)
  line L70 (-291.8044, 402.3487) -> (-291.8044, 477.3487)
  line L71 (-246.5737, 477.267) -> (-291.6933, 477.3339) projected
  line L72 (-291.8044, 477.3487) -> (-246.5737, 477.267)
  line L73 (-243.3598, 554.2673) -> (-243.3598, 481.0972) projected
  line L74 (-246.5737, 477.267) -> (-243.3598, 481.0972)
  line L75 (-243.3598, 481.0972) -> (-243.3598, 554.2673)
  line L76 (-247.2816, 557.3687) -> (-243.3598, 554.2673) projected
  line L77 (-243.3598, 554.2673) -> (-247.2816, 557.3687)
  line L78 (-247.2816, 557.3687) -> (-301.886, 557.3687)
  point P0 (0, 0)
  dimension "d452" = 10
  dimension "d453" = 15
  dimension "d454" = 5
  dimension "d455" = 5
  dimension "d456" = 30
  dimension "d457" = 40
  dimension "d458" = 10
  dimension "d459" = 10
  dimension "d460" = 10
  dimension "d461" = 40
  dimension "d462" = 25
  dimension "d463" = 15
  dimension "d464" = 3
  dimension "d465" = 10
  dimension "d466" = 15
  dimension "d467" = 5
  dimension "d468" = 5
  dimension "d469" = 30
  dimension "d470" = 40
  dimension "d471" = 10
  dimension "d472" = 10
  dimension "d473" = 10
  dimension "d474" = 40
  dimension "d475" = 75
  constraints: 93 end point, 19 collinear, 11 perpendicular, 8 parallel, 4 point on circle, 2 centre point, 1 point on line
  measures "d452" distance of L5.end L7.start
  measures "d453" distance of L7.start L7.end
  measures "d454" distance of L7.end L10.start
  measures "d455" distance of L10.start L10.end
  measures "d456" distance of L10.end L13.end
  measures "d457" distance of L13.end L15.end
  measures "d458" distance of L15.end L17.end
  measures "d459" radius of A0
  measures "d460" distance of L19.start L19.end
  measures "d461" distance of L19.end L21.start
  measures "d462" distance of L0.start L23.start
  measures "d463" distance of L23.start L25.start
  measures "d464" distance of L25.start L27.end
  measures "d465" distance of L27.end L27.start
  measures "d466" distance of L27.start L30.end
  measures "d467" distance of L30.end L30.start
  measures "d468" distance of L30.start L33.end
  measures "d469" distance of L33.end L35.end
  measures "d470" distance of L35.end L37.end
  measures "d471" distance of L37.end L38.end
  measures "d472" radius of A1
  measures "d473" distance of L40.end L40.start
  measures "d474" distance of L40.start L42.start
  measures "d475" distance of L68.start L70.end
extrude "Extrusion34" cut sketch "Sketch44" against normal blind 7
sketch "Sketch45" plane through (291.6933, 477.3339, 0) normal (-0.9999989, -0.0014818, 0) x (0, 0, 1)
  line L0 (7, 0) -> (12, 0) projected
  line L1 (12, 0) -> (7, 0)
  line L2 (7, 0) -> (7, -75)
  line L3 (7, -75) -> (12, -75)
  line L4 (12, -75) -> (12, 0)
  line L5 (7, 0.0147) -> (7, -74.9853) projected
  line L6 (0, 0.0147) -> (0, -74.9853) projected
  line L7 (7, 0.0147) -> (0, 0.0147)
  line L8 (0, 0.0147) -> (0, -74.9853)
  line L9 (0, -74.9853) -> (7, -74.9853)
  line L10 (7, -74.9853) -> (7, 0.0147)
  point P0 (0, -476.9011)
  point P1 (0, 0.0147)
  dimension "d478" = 5
  dimension "d479" = 75
  dimension "d480" = 5
  dimension "d481" = 75
  constraints: 16 end point, 3 equal length, 3 perpendicular, 1 horizontal
  measures "d478" distance of L0.end L0.start
  measures "d479" distance of L0.start L2.end
  measures "d480" distance of L2.end L3.end
  measures "d481" distance of L3.end L0.end
extrude "Extrusion35" cut sketch "Sketch45" against normal blind 7 contours L2 L9 L6 L7 L5
sketch "Sketch46" plane through (246.5737, 477.267, 0) normal (0.0014818, -0.9999989, 0) x (0.9999989, 0.0014818, 0)
  line L0 (0, 7) -> (0, 12) projected
  line L1 (0, 0) -> (45.1196, 0) projected
  line L2 (0, 7) -> (45.1196, 7)
  line L3 (45.1196, 7) -> (45.1196, 0)
  line L4 (45.1196, 0) -> (0, 0)
  line L5 (0, 0) -> (0, 7)
  point P0 (-247.2806, 0)
  constraints: 8 end point, 2 parallel, 1 horizontal, 1 perpendicular
extrude "Extrusion36" cut sketch "Sketch46" against normal blind 7
sketch "Sketch47" plane through (405.5007, 612.3648, 12) normal (0, 1, 0) x (1, 0, 0)
  line L0 (10, 5) -> (13.4296, 5) projected
  line L1 (0, 12) -> (0, 5) projected
  line L2 (10, 5) -> (0, 5)
  line L3 (0, 5) -> (0, 12)
  line L4 (0, 12) -> (10, 12)
  line L5 (10, 12) -> (10, 5)
  point P0 (-405.5007, 12)
  constraints: 8 end point, 2 parallel, 1 horizontal, 1 perpendicular
extrude "Extrusion37" cut sketch "Sketch47" against normal blind 7
body "Solid4"
